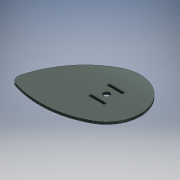
# Autodesk Inventor part: leva00
Saved by Autodesk Inventor 2016 (Build 200138000, 138)
## iProperties
Created: 2016-09-20
Part Number: leva00
Material: Madera (abedul)
Document SubType Name: Modeling
Designer: i95sa
Density: 0.55 g/cm^3
Appearance: Gris plomo - Pulido
Author: i95sa
Autodesk Inventor part; units mm, degrees
ref_plane "YZ Plane" through (0, 0, 0) normal (1, 0, 0) x (0, 1, 0)
ref_plane "XZ Plane" through (0, 0, 0) normal (0, 1, 0) x (-1, 0, 0)
ref_plane "XY Plane" through (0, 0, 0) normal (0, 0, 1) x (1, 0, 0)
sketch "Boceto1" plane through (0, 0, 0) normal (0, 0, 1) x (1, 0, 0)
  arc A0 (47.3907, 26.0532) -> (-47.3907, -26.0532) centre (0, 0) ccw
  arc A1 (-72.9305, -40.0939) -> (-94.8031, -52.1185) centre (-83.8668, -46.1062) ccw
  line L0 (-97.9695, -53.8592) -> (-103.9817, -42.9229)
  line L1 (-25.49, 47.696) -> (-35.5105, 65.9231)
  line L2 (-35.5105, 65.9231) -> (-103.9817, -42.9229)
  line L3 (-103.9817, -42.9229) -> (-77.4008, -0.6682)
  arc A2 (-25.49, 47.696) -> (-77.4008, -0.6682) centre (39.7379, -74.3561) ccw
  arc A3 (-77.4008, -0.6682) -> (-95.9085, -42.8278) centre (54.8753, -83.8785) ccw
  line L4 (3.6454, 2.0041) -> (47.3907, 26.0532)
  line L5 (-3.6454, -2.0041) -> (-97.9695, -53.8592)
  arc A4 (-47.3907, -26.0532) -> (47.3907, 26.0532) centre (0, 0) ccw
  arc A5 (-94.8031, -52.1185) -> (-72.9305, -40.0939) centre (-83.8668, -46.1062) ccw
  line L6 (-97.9695, -53.8592) -> (-91.9572, -64.7955)
  line L7 (26.6128, -47.0787) -> (36.6333, -65.3059)
  line L8 (36.6333, -65.3059) -> (-91.9572, -64.7955)
  line L9 (-91.9572, -64.7955) -> (-42.0376, -64.9936)
  arc A6 (-42.0376, -64.9936) -> (26.6128, -47.0787) centre (-41.4883, 73.3938) ccw
  arc A7 (-87.5511, -58.0299) -> (-42.0376, -64.9936) centre (-41.4173, 91.2771) ccw
  dimension "d0" = 108.16
  dimension "d6" = 24.96
  dimension "d7" = 12.48
  dimension "d8" = 20.8
  dimension "d9" = 49.92
  constraints: 20 end point, 20 point on circle, 8 centre point, 6 symmetric about line, 5 point on line, 4 tangent, 1 collinear, 4 other
  measures "d0" diameter of A0
  measures "d6" diameter of A1
  measures "d7" distance of L0.start L0.end
  measures "d8" distance of L1.start L1.end
  measures "d9" distance of L0.end L3.end
extrude "Extrusión2" add sketch "Boceto1" along normal blind 4 contours A4 A0 | A0 L5 A1 A3 A2 | A6 A7 A5 L5 A4 | L5 A1 | A5 L5
sketch "Boceto2" plane through (0, 0, 4) normal (0, 0, 1) x (1, 0, 0)
  line L0 (0, 0) -> (0, 12.5)
  line L1 (0, 12.5) -> (-12.5, 12.5)
  line L2 (-12.5, 12.5) -> (-12.5, 16.7)
  line L3 (-12.5, 16.7) -> (12.5, 16.7)
  line L4 (12.5, 16.7) -> (12.5, 12.5)
  line L5 (12.5, 12.5) -> (0, 12.5)
  line L6 (0, 0) -> (12.5, 0)
  line L7 (0, 0) -> (0, -12.5)
  line L8 (0, -12.5) -> (-12.5, -12.5)
  line L9 (-12.5, -12.5) -> (-12.5, -16.7)
  line L10 (-12.5, -16.7) -> (12.5, -16.7)
  line L11 (12.5, -16.7) -> (12.5, -12.5)
  line L12 (12.5, -12.5) -> (0, -12.5)
  circle A0 centre (0, 0) radius 5
  dimension "d24" = 12.5
  dimension "d25" = 12.5
  dimension "d26" = 4.2
  dimension "d27" = 25
  dimension "d28" = 10
  constraints: 26 end point, 5 perpendicular, 5 symmetric about line, 3 point on line, 1 centre point, 1 coincident, 1 parallel, 1 vertical
  measures "d24" distance of L0.start L0.end
  measures "d25" distance of L0.end L1.end
  measures "d26" distance of L1.end L2.end
  measures "d27" distance of L2.end L3.end
  measures "d28" diameter of A0
extrude "Extrusión3" cut sketch "Boceto2" against normal blind 4
